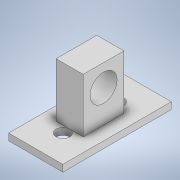
# Autodesk Inventor part: Main Axle notch
Saved by Autodesk Inventor 2020 (Build 240168000, 168)
## iProperties
Created: 2021-01-30
Part Number: Main Axle notch
Material: Generic
Document SubType Name: Modeling
Designer: magda
Density: 1 g/cm^3
Appearance: Default
Author: magda
Autodesk Inventor part; units mm, degrees
ref_plane "YZ Plane" through (0, 0, 0) normal (1, 0, 0) x (0, 1, 0)
ref_plane "XZ Plane" through (0, 0, 0) normal (0, 1, 0) x (-1, 0, 0)
ref_plane "XY Plane" through (0, 0, 0) normal (0, 0, 1) x (1, 0, 0)
sketch "Sketch1" plane through (0, 0, 0) normal (0, 1, 0) x (-1, 0, 0)
  line L0 (18.4951, 35.5107) -> (-6.9049, 35.5107)
  line L1 (-6.9049, 35.5107) -> (-6.9049, -15.2893)
  line L2 (-6.9049, -15.2893) -> (18.4951, -15.2893)
  line L3 (18.4951, -15.2893) -> (18.4951, 35.5107)
  point P0 (0, 0)
  dimension "d0" = 50.8
  dimension "d1" = 25.4
  constraints: 8 end point, 2 parallel, 1 horizontal, 1 perpendicular
  measures "d0" distance of L0.end L1.end
  measures "d1" distance of L1.end L2.end
extrude "Extrusion1" add sketch "Sketch1" along normal blind 3.175
sketch "Sketch2" plane through (0, 3.175, 0) normal (0, 1, 0) x (1, 0, 0)
  line L0 (-18.4951, 15.2893) -> (-18.4951, -35.5107) projected
  line L1 (6.9049, 15.2893) -> (-18.4951, 15.2893) projected
  point P0 (0, 0)
  point P1 (-5.7951, -22.8107)
  point P2 (-5.7951, 2.5893)
  dimension "d4" = 12.7
  dimension "d5" = 12.7
  dimension "d6" = 25.4
  dimension "d7" = 12.7
  measures "d4" distance from line of point (-5.795, 2.589) L0
  measures "d5" distance from line of point (-5.795, -22.811) L0
  measures "d6" distance of point (-5.795, 2.589) point (-5.795, -22.811)
  measures "d7" distance from line of L1 point (-5.795, 2.589)
hole "Hole1" at (-5.7951, 3.175, 22.8107) at (-5.7951, 3.175, -2.5893) direction (0, -1, 0) diameter 6.35 end through all
sketch "Sketch3" plane through (0, 3.175, 0) normal (0, 1, 0) x (1, 0, 0)
  line L0 (-12.1451, -19.6357) -> (0.5549, -19.6357)
  line L1 (0.5549, -19.6357) -> (0.5549, -0.5857)
  line L2 (0.5549, -0.5857) -> (-12.1451, -0.5857)
  line L3 (-12.1451, -0.5857) -> (-12.1451, -19.6357)
  line L4 (-18.4951, 15.2893) -> (-18.4951, -35.5107) projected
  line L5 (6.9049, 15.2893) -> (-18.4951, 15.2893) projected
  line L6 (-18.4951, -35.5107) -> (6.9049, -35.5107) projected
  point P0 (0, 0)
  dimension "d15" = 12.7
  dimension "d16" = 6.35
  dimension "d17" = 15.875
  dimension "d18" = 15.875
  constraints: 8 end point, 2 parallel, 1 horizontal, 1 perpendicular
  measures "d15" distance of L2.end L1.end
  measures "d16" distance between parallel lines of L3 L4
  measures "d17" distance between parallel lines of L5 L2
  measures "d18" distance between parallel lines of L6 L0
extrude "Extrusion2" add sketch "Sketch3" along normal blind 25.4
sketch "Sketch4" plane through (0.5549, 3.175, 19.6357) normal (1, 0, 0) x (0, 0, -1)
  circle A0 centre (9.525, 15.24) radius 6.35
  line L0 (19.05, 0) -> (19.05, 25.4) projected
  line L1 (0, 25.4) -> (19.05, 25.4) projected
  point P0 (19.6357, -3.175)
  dimension "d21" = 9.525
  dimension "d22" = 12.7
  dimension "d23" = 10.16
  constraints: 1 centre point
  measures "d21" distance from line of L0 A0.centre
  measures "d22" diameter of A0
  measures "d23" distance from line of L1 A0.centre
extrude "Extrusion3" cut sketch "Sketch4" against normal blind 25.4
body "Solid1"
